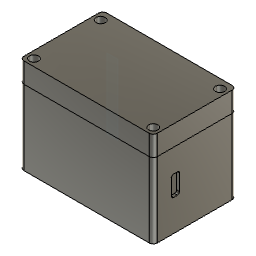
ESP32 Tally Case (Autodesk Fusion 360 design; units mm, degrees)
Autodesk Fusion 360 part; units mm, degrees
sketch "Sketch1" plane through (0, 0, 0) normal (0, 0, 1) x (1, 0, 0)
  line L0 (0, 0) -> (62, 0)
  line L1 (62, 0) -> (62, 39)
  line L2 (62, 39) -> (0, 39)
  line L3 (0, 39) -> (0, 0)
  line L4 (0, 0) -> (5, 0) construction
  line L5 (5, 0) -> (5, 5) construction
  line L6 (5, 5) -> (0, 5) construction
  line L7 (0, 5) -> (0, 0) construction
  line L8 (5, 5) -> (57, 5)
  line L9 (57, 5) -> (57, 34)
  line L10 (57, 34) -> (5, 34)
  line L11 (5, 34) -> (5, 5)
  dimension "d3" = 39
  dimension "d4" = 62
  dimension "d5" = 5
  dimension "d6" = 5
  dimension "d7" = 52
  dimension "d8" = 29
  constraint horizontal L0
  constraint vertical L1
  constraint horizontal L2
  constraint vertical L3
  constraint coincident L0.start L3.end
  constraint horizontal L4
  constraint vertical L5
  constraint horizontal L6
  constraint vertical L7
  constraint horizontal L8
  constraint vertical L9
  constraint horizontal L10
  constraint vertical L11
  measures "d3" distance of L0.start L2.end
  measures "d4" distance of L0.start L0.end
  measures "d5" distance of L0.start L4.end
  measures "d6" distance of L0.start L6.end
  measures "d7" distance of L5.end L8.end
  measures "d8" distance of L5.end L10.end
extrude "Extrude1" add sketch "Sketch1" along normal blind 8 contours L0 L1 L2 L3 | L8 L9 L10 L11 makes body 1
extrude "Extrude2" add sketch "Sketch1" along normal blind 23 bodies 1
sketch "Sketch2" plane through (0, 0, 23) normal (0, 0, 1) x (-1, 0, 0)
  line L0 (-5, -5) -> (-5, -34)
  line L1 (-5, -34) -> (-57, -34)
  line L2 (-57, -34) -> (-57, -5)
  line L3 (-57, -5) -> (-5, -5)
  line L4 (0, -39) -> (0, 0)
  line L5 (0, 0) -> (-62, 0)
  line L6 (-62, 0) -> (-62, -39)
  line L7 (-62, -39) -> (0, -39)
  line L8 (-31, -34) -> (-10.5, -34)
  line L9 (-31, -34) -> (-51.5, -34)
  line L10 (-62, -39) -> (-62, -37) construction
  line L11 (-62, -37) -> (0, -37) construction
  line L12 (-51.5, -34) -> (-10.5, -34)
  line L13 (-10.5, -34) -> (-10.5, -37)
  line L14 (-10.5, -37) -> (-51.5, -37)
  line L15 (-51.5, -37) -> (-51.5, -34)
  dimension "d13" = 20.5
  dimension "d14" = 20.5
  dimension "d15" = 2
  constraint midpoint L1 L8.start
  constraint parallel L1 L8
  constraint parallel L1 L9
  constraint coincident L6.end L7.start
  constraint perpendicular L7 L10
  constraint coincident L4 L11.end
  constraint perpendicular L4 L11
  constraint horizontal L12
  constraint vertical L13
  constraint horizontal L14
  constraint vertical L15
  constraint coincident L11 L13.end
  measures "d13" distance of L8.start L8.end
  measures "d14" distance of L8.start L9.end
  measures "d15" distance of L6.end L10.end
extrude "Extrude3" add sketch "Sketch2" along normal blind 6 bodies 1
sketch "Sketch3" plane through (0, 0, 29) normal (0, 0, 1) x (-1, 0, 0)
  line L0 (-10.5, -37) -> (-51.5, -37)
  line L1 (-51.5, -37) -> (-51.5, -34)
  line L2 (-51.5, -34) -> (-57, -34)
  line L3 (-57, -34) -> (-57, -5)
  line L4 (-57, -5) -> (-5, -5)
  line L5 (-5, -5) -> (-5, -34)
  line L6 (-5, -34) -> (-10.5, -34)
  line L7 (-10.5, -34) -> (-10.5, -37)
  line L8 (-62, -39) -> (0, -39)
  line L9 (0, -39) -> (0, 0)
  line L10 (0, 0) -> (-62, 0)
  line L11 (-62, 0) -> (-62, -39)
  line L12 (-51.5, -37) -> (-51.5, -39)
  line L13 (-10.5, -37) -> (-10.5, -39)
  constraint coincident L0.end L1.start
  constraint coincident L8 L12.end
  constraint perpendicular L8 L12
  constraint coincident L0.start L7.end
  constraint coincident L8 L13.end
  constraint perpendicular L8 L13
extrude "Extrude4" add sketch "Sketch3" along normal blind 29 contours L1 L2 L3 L4 L5 L6 L7 L8 L9 L10 L11 L12 L13 bodies 1
sketch "Sketch4" plane through (51.5, 0, 0) normal (-1, 0, 0) x (0, -1, 0)
  line L0 (-37, 23) -> (-34, 23)
  line L1 (-34, 23) -> (-34, 58)
  line L2 (-34, 58) -> (-39, 58)
  line L3 (-39, 58) -> (-39, 29)
  line L4 (-39, 29) -> (-37, 29)
  line L5 (-37, 29) -> (-37, 23)
  line L6 (-37, 29) -> (-37, 58)
  constraint coincident L4.end L5.start
  constraint coincident L2 L6.end
  constraint perpendicular L2 L6
sketch "Sketch5" plane through (10.5, 0, 0) normal (1, 0, 0) x (0, 1, 0)
  line L0 (34, 23) -> (37, 23)
  line L1 (37, 23) -> (37, 29)
  line L2 (37, 29) -> (39, 29)
  line L3 (39, 29) -> (39, 58)
  line L4 (39, 58) -> (34, 58)
  line L5 (34, 58) -> (34, 23)
  line L6 (37, 29) -> (37, 58)
  constraint coincident L1.end L2.start
  constraint coincident L4 L6.end
  constraint perpendicular L4 L6
extrude "Extrude5" add sketch "Sketch4" along normal blind 2.5 contours L2 L3 L4 L6 bodies 1
extrude "Extrude6" add sketch "Sketch5" along normal blind 2.5 contours L2 L3 L4 L6 bodies 1
extrude "Extrude7" add 1 faces at (20.6667, 0, 19.3333) along direction (0, -1, 0) blind 2 on bodies 1 bodies 1
extrude "Extrude8" add 1 faces at (62, 25.3333, 38.6667) along direction (1, 0, 0) blind 2 on bodies 1 bodies 1
extrude "Extrude9" add 1 faces at (0, 25.3333, 38.6667) along direction (-1, 0, 0) blind 2 on bodies 1 bodies 1
ref_plane "WorkPlane1" through (0, 0, 23) normal (0, 0, 1) x (1, 0, 0)
split "Split1" by plane through (0, 0, 23) normal (0, 0, 1) bodies 1 makes body 2 at (42, -2, 46.3333)
extrude "Extrude10" add 1 faces at (37, 38.3333, 29) along direction (0, 0, 1) blind 5 on bodies 2 bodies 2
sketch "Sketch6" plane through (13, 0, 0) normal (1, 0, 0) x (0, 1, 0)
  line L0 (37, 34) -> (39, 34)
  line L1 (39, 34) -> (39, 58)
  line L2 (39, 58) -> (37, 58)
  line L3 (37, 58) -> (37, 34)
  line L4 (37, 58) -> (39, 58)
  line L5 (39, 58) -> (39, 51)
  line L6 (39, 51) -> (37, 51)
  line L7 (37, 51) -> (37, 58)
  dimension "d33" = 7
  constraint horizontal L4
  constraint vertical L5
  constraint horizontal L6
  constraint vertical L7
  constraint coincident L2.end L3.start
  measures "d33" distance of L2.end L6.end
extrude "Extrude11" add sketch "Sketch6" along normal blind 40 contours L1 L2 L3 L4 L5 L6 L7 bodies 2
sketch "Sketch7" plane through (0, 34, 0) normal (0, -1, 0) x (1, 0, 0)
  line L0 (5, 23) -> (10.5, 23)
  line L1 (10.5, 23) -> (10.5, 58)
  line L2 (10.5, 58) -> (5, 58)
  line L3 (5, 58) -> (5, 23)
move_body "Move1" bodies 2 to x (1, 0, 0) y (0, 1, 0) z (0, 0, 1) at (0, 0, 2)
extrude "Extrude12" add 1 faces at (39.6667, 0.3333, 25) along direction (0, 0, -1) blind 2 on bodies 2 bodies 2
sketch "Sketch8" plane through (10.5, 0, 0) normal (1, 0, 0) x (0, 1, 0)
  line L0 (37, 23) -> (37, 60)
  line L1 (37, 60) -> (34, 60)
  line L2 (34, 60) -> (34, 23)
  line L3 (34, 23) -> (37, 23)
  line L4 (34, 23) -> (37, 23)
  line L5 (37, 23) -> (37, 25)
  line L6 (37, 25) -> (34, 25)
  line L7 (34, 25) -> (34, 23)
  dimension "d38" = 2
  constraint horizontal L4
  constraint vertical L5
  constraint horizontal L6
  constraint vertical L7
  measures "d38" distance of L2.end L6.end
extrude "Extrude13" add sketch "Sketch8" along normal blind 41 contours L0 L2 L3 L4 L5 L6 L7 bodies 2
sketch "Sketch9" plane through (0, 34, 0) normal (0, -1, 0) x (1, 0, 0)
  line L0 (10.5, 25) -> (10.5, 60)
  line L1 (10.5, 60) -> (5, 60)
  line L2 (5, 60) -> (5, 23)
  line L3 (5, 23) -> (57, 23)
  line L4 (57, 23) -> (57, 60)
  line L5 (57, 60) -> (51.5, 60)
  line L6 (51.5, 60) -> (51.5, 25)
  line L7 (51.5, 25) -> (10.5, 25)
extrude "Extrude14" add sketch "Sketch9" along normal blind 2 bodies 2
extrude "Extrude15" add 1 faces at (55.1667, 32, 36) along direction (0, -1, 0) blind 2 on bodies 2 bodies 2
sketch "Sketch10" plane through (0, 0, 25) normal (0, 0, 1) x (-1, 0, 0)
  line L0 (-10.5, -37) -> (-10.5, -30)
  line L1 (-10.5, -30) -> (-51.5, -30)
  line L2 (-51.5, -30) -> (-51.5, -37)
  line L3 (-51.5, -37) -> (-10.5, -37)
  line L4 (-51.5, -30) -> (-10.5, -30)
  line L5 (-10.5, -30) -> (-10.5, -32)
  line L6 (-10.5, -32) -> (-51.5, -32)
  line L7 (-51.5, -32) -> (-51.5, -30)
  dimension "d45" = 41
  dimension "d46" = 2
  constraint horizontal L4
  constraint vertical L5
  constraint horizontal L6
  constraint vertical L7
  constraint coincident L1.end L2.start
  measures "d45" distance of L1.end L0.end
  measures "d46" distance of L1.end L6.end
extrude "Extrude16" add sketch "Sketch10" along normal blind 25 contours L0 L1 L2 L4 L5 L6 L7 bodies 2
extrude "Extrude17" add 2 faces at (22.3333, 0.3333, 60) (37, 38.3333, 60) along direction (0, 0, 1) blind 2 separate body on bodies 2 makes body 3
extrude "Extrude18" cut 2 faces at (55.1667, 30, 61.3333) (8.6667, 30, 60.6667) along direction (0, 1, 0) blind 2 on bodies 3 bodies 3
extrude "Extrude19" add 1 faces at (51.5, 35.3333, 61.3333) along direction (-1, 0, 0) blind 41 on bodies 3 bodies 3
extrude "Extrude20" add 3 faces at (37, 33.6667, 62) (22.3333, 0.3333, 62) (37, 38.3333, 62) along direction (0, 0, 1) blind 6 on bodies 3 bodies 3
sketch "Sketch11" plane through (0, 0, 68) normal (0, 0, 1) x (-1, 0, 0)
  line L0 (-64, -39) -> (2, -39)
  line L1 (2, -39) -> (2, 2)
  line L2 (2, 2) -> (-64, 2)
  line L3 (-64, 2) -> (-64, -39)
  line L4 (-5, -32) -> (-57, -32)
  line L5 (-57, -32) -> (-57, -5)
  line L6 (-57, -5) -> (-5, -5)
  line L7 (-5, -5) -> (-5, -32)
  line L8 (-5, -32) -> (-5, -39) construction
  line L9 (-5, -5) -> (-5, 2) construction
  line L10 (-5, -5) -> (2, -5) construction
  line L11 (-57, -5) -> (-57, 2) construction
  line L12 (-57, -5) -> (-64, -5) construction
  line L13 (-57, -32) -> (-64, -32) construction
  line L14 (-57, -32) -> (-57, -39) construction
  line L15 (-5, -32) -> (2, -32) construction
  line L16 (-5, 2) -> (-7, 2) construction
  line L17 (-57, 2) -> (-55, 2) construction
  line L18 (-5, 2) -> (-5, 0) construction
  line L19 (-5, -39) -> (-5, -37) construction
  line L20 (-55, 2) -> (-55, 0) construction
  line L21 (-5, -37) -> (-7, -37)
  line L22 (-7, -37) -> (-55, -37)
  line L23 (-55, -37) -> (-55, 0)
  line L24 (-55, 0) -> (-7, 0)
  line L25 (-7, 0) -> (-7, -37)
  line L26 (-64, -5) -> (-62, -5) construction
  line L27 (-62, -5) -> (-62, -7) construction
  line L28 (-62, -7) -> (-64, -7) construction
  line L29 (-64, -7) -> (-64, -5) construction
  line L30 (2, -32) -> (0, -32)
  line L31 (0, -32) -> (0, -30)
  line L32 (0, -30) -> (2, -30)
  line L33 (2, -30) -> (2, -32)
  line L34 (0, -30) -> (-62, -30)
  line L35 (-62, -30) -> (-62, -7)
  line L36 (-62, -7) -> (0, -7)
  line L37 (0, -7) -> (0, -30)
  dimension "d57" = 2
  dimension "d58" = 2
  dimension "d59" = 2
  dimension "d60" = 2
  dimension "d61" = 2
  dimension "d62" = 2
  dimension "d63" = 2
  dimension "d64" = 2
  dimension "d65" = 2
  dimension "d66" = 2
  constraint coincident L4.start L7.end
  constraint coincident L0 L8.end
  constraint perpendicular L0 L8
  constraint coincident L6.end L7.start
  constraint coincident L2 L9.end
  constraint perpendicular L2 L9
  constraint coincident L1 L10.end
  constraint perpendicular L1 L10
  constraint coincident L5.end L6.start
  constraint coincident L2 L11.end
  constraint perpendicular L2 L11
  constraint coincident L3 L12.end
  constraint perpendicular L3 L12
  constraint coincident L4.end L5.start
  constraint coincident L3 L13.end
  constraint perpendicular L3 L13
  constraint coincident L0 L14.end
  constraint perpendicular L0 L14
  constraint coincident L1 L15.end
  constraint perpendicular L1 L15
  constraint perpendicular L9 L16
  constraint perpendicular L11 L17
  constraint perpendicular L16 L18
  constraint perpendicular L0 L19
  constraint perpendicular L17 L20
  constraint perpendicular L19 L21
  constraint horizontal L22
  constraint vertical L23
  constraint horizontal L24
  constraint vertical L25
  constraint horizontal L26
  constraint vertical L27
  constraint horizontal L28
  constraint vertical L29
  constraint horizontal L30
  constraint vertical L31
  constraint horizontal L32
  constraint vertical L33
  constraint horizontal L34
  constraint vertical L35
  constraint horizontal L36
  constraint vertical L37
  measures "d57" distance of L9.end L16.end
  measures "d58" distance of L11.end L17.end
  measures "d59" distance of L9.end L18.end
  measures "d60" distance of L8.end L19.end
  measures "d61" distance of L17.end L20.end
  measures "d62" distance of L19.end L21.end
  measures "d63" distance of L12.end L26.end
  measures "d64" distance of L12.end L28.end
  measures "d65" distance of L15.end L30.end
  measures "d66" distance of L15.end L32.end
extrude "Extrude21" cut sketch "Sketch11" against normal blind 22 contours L7 L34 L36 L37 | L4 L22 L23 L25 | L6 L23 L24 L25 | L5 L34 L35 L36 bodies 3
sketch "Sketch12" plane through (0, 37, 0) normal (0, -1, 0) x (1, 0, 0)
  line L0 (7, 60) -> (55, 60)
  line L1 (55, 60) -> (55, 68)
  line L2 (55, 68) -> (7, 68)
  line L3 (7, 68) -> (7, 60)
  line L4 (31, 60) -> (27, 60)
  line L5 (31, 60) -> (35, 60)
  line L6 (35, 60) -> (27, 60)
  line L7 (27, 60) -> (27, 61)
  line L8 (27, 61) -> (35, 61)
  line L9 (35, 61) -> (35, 60)
  dimension "d69" = 4
  dimension "d70" = 4
  dimension "d71" = 8
  dimension "d72" = 1
  constraint midpoint L0 L4.start
  constraint parallel L0 L4
  constraint parallel L0 L5
  constraint horizontal L6
  constraint vertical L7
  constraint horizontal L8
  constraint vertical L9
  measures "d69" distance of L4.start L4.end
  measures "d70" distance of L4.start L5.end
  measures "d71" distance of L5.end L4.end
  measures "d72" distance of L5.end L8.end
extrude "Extrude22" add sketch "Sketch12" along normal blind 37 contours L0 L4 L5 L6 L7 L8 L9 bodies 3
sketch "Sketch13" plane through (0, 0, 68) normal (0, 0, 1) x (-1, 0, 0)
  line L0 (-57, -30) -> (-62, -30)
  line L1 (-62, -30) -> (-62, -7)
  line L2 (-62, -7) -> (-57, -7)
  line L3 (-57, -7) -> (-57, -5)
  line L4 (-57, -5) -> (-55, -5)
  line L5 (-55, -5) -> (-55, 0)
  line L6 (-55, 0) -> (-7, 0)
  line L7 (-7, 0) -> (-7, -5)
  line L8 (-7, -5) -> (-5, -5)
  line L9 (-5, -5) -> (-5, -7)
  line L10 (-5, -7) -> (0, -7)
  line L11 (0, -7) -> (0, -30)
  line L12 (0, -30) -> (-5, -30)
  line L13 (-5, -30) -> (-5, -32)
  line L14 (-5, -32) -> (-7, -32)
  line L15 (-7, -32) -> (-7, -37)
  line L16 (-7, -37) -> (-55, -37)
  line L17 (-55, -37) -> (-55, -32)
  line L18 (-55, -32) -> (-57, -32)
  line L19 (-57, -32) -> (-57, -30)
  line L20 (-64, -39) -> (2, -39)
  line L21 (2, -39) -> (2, 2)
  line L22 (2, 2) -> (-64, 2)
  line L23 (-64, 2) -> (-64, -39)
extrude "Extrude23" add sketch "Sketch13" along normal blind 2 contours L0 L1 L2 L3 L4 L5 L6 L7 L8 L9 L10 L11 L12 L13 L14 L15 L16 L17 L18 L19 | L20 L21 L22 L23 bodies 3
sketch "Sketch14" plane through (0, 0, 23) normal (0, 0, -1) x (1, 0, 0)
  line L0 (57, -5) -> (57, -30)
  line L1 (57, -30) -> (5, -30)
  line L2 (5, -30) -> (5, -5)
  line L3 (5, -5) -> (57, -5)
  line L4 (64, -39) -> (64, 2)
  line L5 (64, 2) -> (-2, 2)
  line L6 (-2, 2) -> (-2, -39)
  line L7 (-2, -39) -> (64, -39)
  line L8 (64, -39) -> (57, -30) construction
  line L9 (64, 2) -> (57, -5) construction
  line L10 (5, -30) -> (-2, -39) construction
  line L11 (-2, 2) -> (5, -5) construction
  circle A0 centre (1.5, -34.5) radius 2.25
  circle A1 centre (1.5, -1.5) radius 2.25
  circle A2 centre (60.5, -1.5) radius 2.25
  circle A3 centre (60.5, -34.5) radius 2.25
  dimension "d77" = 4.5
  dimension "d78" = 4.5
  dimension "d79" = 4.5
  dimension "d80" = 4.5
  constraint coincident L4.start L7.end
  constraint coincident L0.end L1.start
  constraint coincident L4.end L5.start
  constraint coincident L0.start L3.end
  constraint coincident L1.end L2.start
  constraint coincident L6.end L7.start
  constraint coincident L5.end L6.start
  constraint coincident L2.end L3.start
  constraint midpoint L10 A0.centre
  constraint midpoint L11 A1.centre
  constraint midpoint L9 A2.centre
  constraint midpoint L8 A3.centre
  measures "d77" diameter of A0
  measures "d78" diameter of A1
  measures "d79" diameter of A2
  measures "d80" diameter of A3
extrude "Extrude24" cut sketch "Sketch14" along normal blind 25 and the other way blind 50 contours A0 | A1 | A2 | A3 bodies 1 2 3
fillet "Fillet1" radius 2 12 edges at (64, 39, 11.5) (64, -2, 11.5) (-2, 39, 11.5) (-2, -2, 11.5) (64, 39, 41.5) (64, -2, 41.5) (-2, 39, 41.5) (-2, -2, 41.5) (64, 39, 65) (64, -2, 65) (-2, 39, 65) (-2, -2, 65) on bodies 1 2 3
sketch "Sketch15" plane through (0, 0, 0) normal (0, 0, -1) x (1, 0, 0)
  arc A0 (0, 2) -> (-2, 0) centre (0, 0) ccw
  line L0 (-2, 0) -> (-2, -37)
  arc A1 (-2, -37) -> (0, -39) centre (0, -37) ccw
  line L1 (0, -39) -> (62, -39)
  arc A2 (62, -39) -> (64, -37) centre (62, -37) ccw
  line L2 (64, -37) -> (64, 0)
  arc A3 (64, 0) -> (62, 2) centre (62, 0) ccw
  line L3 (62, 2) -> (0, 2)
  circle A4 centre (60.5, -1.5) radius 2.25
  circle A5 centre (1.5, -34.5) radius 2.25
  circle A6 centre (60.5, -34.5) radius 2.25
  circle A7 centre (1.5, -1.5) radius 2.25
  line L4 (31, -39) -> (31, 2)
  line L5 (38.5, -11) -> (23.5, -11) construction
  line L6 (23.5, -11) -> (23.5, -26) construction
  line L7 (23.5, -26) -> (38.5, -26) construction
  line L8 (38.5, -26) -> (38.5, -11) construction
  line L9 (38.5, -11) -> (23.5, -26) construction
  line L10 (23.5, -11) -> (38.5, -26) construction
  line L11 (31, -18.5) -> (38.5, -26) construction
  line L12 (23.5, -11) -> (31, -18.5) construction
  circle A8 centre (27.25, -14.75) radius 2.25
  circle A9 centre (34.75, -22.25) radius 2.25
  point P0 (31, -18.5)
  dimension "d87" = 15
  dimension "d88" = 15
  dimension "d90" = 4.5
  dimension "d91" = 4.5
  constraint midpoint L1 L4.start
  constraint midpoint L3 L4.end
  constraint horizontal L5
  constraint perpendicular L5 L6
  constraint parallel L5 L7
  constraint parallel L6 L8
  constraint coincident L9 P0
  constraint coincident L10 P0
  constraint midpoint L4 P0
  constraint coincident P0 L11.start
  constraint midpoint L12 A8.centre
  constraint midpoint L11 A9.centre
  measures "d87" distance of L6.end L7.end
  measures "d88" distance of L5.end L6.end
  measures "d90" diameter of A8
  measures "d91" diameter of A9
extrude "Extrude25" cut sketch "Sketch15" against normal blind 4 contours A8 | A9 bodies 1
sketch "Sketch16" plane through (5, 0, 0) normal (1, 0, 0) x (0, 1, 0)
  line L0 (34, 23) -> (5, 23)
  line L1 (5, 23) -> (5, 8)
  line L2 (5, 8) -> (34, 8)
  line L3 (34, 8) -> (34, 23)
  line L4 (19.5, 8) -> (12, 8)
  line L5 (19.5, 8) -> (27, 8)
  line L6 (12, 8) -> (27, 8)
  line L7 (27, 8) -> (27, 16)
  line L8 (27, 16) -> (12, 16)
  line L9 (12, 16) -> (12, 8)
  dimension "d94" = 7.5
  dimension "d95" = 7.5
  dimension "d96" = 8
  constraint midpoint L2 L4.start
  constraint parallel L2 L4
  constraint parallel L2 L5
  constraint horizontal L6
  constraint vertical L7
  constraint horizontal L8
  constraint vertical L9
  measures "d94" distance of L4.start L4.end
  measures "d95" distance of L4.start L5.end
  measures "d96" distance of L4.end L8.end
extrude "Extrude26" cut sketch "Sketch16" against normal blind 36 contours L2 L4 L5 L6 L7 L8 L9 bodies 1
fillet "Fillet2" radius 2.5 4 edges at (1.5, 27, 8) (1.5, 12, 8) (1.5, 12, 16) (1.5, 27, 16) on bodies 1
fillet "Fillet3" radius 1.5 8 edges at (-2, 12.7322, 15.2678) (-2, 12, 12) (-2, 12.7322, 8.7322) (-2, 19.5, 8) (-2, 26.2678, 8.7322) (-2, 27, 12) (-2, 26.2678, 15.2678) (-2, 19.5, 16) on bodies 1
extrude "Extrude27" cut 1 faces at (57, 24.3333, 13) along direction (1, 0, 0) blind 0.5 on bodies 1 bodies 1
extrude "Extrude28" cut 1 faces at (5, 17.8333, 20.6667) along direction (-1, 0, 0) blind 0.5 on bodies 1 bodies 1
extrude "Extrude29" cut 1 faces at (39.8333, 34, 13) along direction (0, 1, 0) blind 0.5 on bodies 1 bodies 1
extrude "Extrude30" cut 1 faces at (39.8333, 5, 18) along direction (0, -1, 0) blind 0.5 on bodies 1 bodies 1
extrude "Extrude31" cut 1 faces at (10.5, 35.3333, 45) along direction (-1, 0, 0) blind 0.5 on bodies 2 bodies 2
extrude "Extrude32" cut 1 faces at (51.5, 35.3333, 45) along direction (1, 0, 0) blind 0.5 on bodies 2 bodies 2
extrude "Extrude33" cut 1 faces at (38, 32, 33.3333) along direction (0, -1, 0) blind 0.5 on bodies 2 bodies 2
copy_body "Body->Comp1" bodies 3 removing the originals makes body 4 in component "Component"
copy_body "Body->Comp2" bodies 2 removing the originals makes body 5 in component "Component'"
extrude "Extrude1'" add 1 faces at (38, 31.5, 33.3333) along direction (0, 1, 0) blind 0.5 on bodies 5 bodies 5 in component "Component'"
sketch "Sketch17" plane through (0, 0, 36) normal (0, 0, 1) x (-1, 0, 0)
  line L0 (-13, -39) -> (-13, -37)
  line L1 (-13, -37) -> (-49, -37)
  line L2 (-49, -37) -> (-49, -39)
  line L3 (-49, -39) -> (-13, -39)
  line L4 (-31, -39) -> (-46, -39)
  line L5 (-31, -39) -> (-16, -39)
  line L6 (-16, -39) -> (-13, -39)
  line L7 (-13, -39) -> (-13, -37)
  line L8 (-13, -37) -> (-16, -37)
  line L9 (-16, -37) -> (-16, -39)
  line L10 (-46, -39) -> (-49, -39)
  line L11 (-49, -39) -> (-49, -37)
  line L12 (-49, -37) -> (-46, -37)
  line L13 (-46, -37) -> (-46, -39)
  dimension "d119" = 15
  dimension "d120" = 15
  constraint midpoint L3 L4.start
  constraint parallel L3 L4
  constraint parallel L3 L5
  constraint horizontal L6
  constraint vertical L7
  constraint horizontal L8
  constraint vertical L9
  constraint coincident L0.end L1.start
  constraint horizontal L10
  constraint vertical L11
  constraint horizontal L12
  constraint vertical L13
  constraint coincident L1.end L2.start
  measures "d119" distance of L4.start L4.end
  measures "d120" distance of L4.start L5.end
extrude "Extrude2'" add sketch "Sketch17" along normal blind 17 contours L0 L1 L3 L6 L7 L8 L9 | L1 L2 L3 L10 L11 L12 L13 bodies 5 in component "Component'"
sketch "Sketch18" plane through (0, 5, 0) normal (0, 1, 0) x (-1, 0, 0)
  line L0 (-5, 23) -> (-5, 60)
  line L1 (-5, 60) -> (-57, 60)
  line L2 (-57, 60) -> (-57, 23)
  line L3 (-57, 23) -> (-5, 23)
  line L4 (-57, 23) -> (-5, 23)
  line L5 (-5, 23) -> (-5, 29)
  line L6 (-5, 29) -> (-57, 29)
  line L7 (-57, 29) -> (-57, 23)
  dimension "d123" = 6
  constraint horizontal L4
  constraint vertical L5
  constraint horizontal L6
  constraint vertical L7
  constraint coincident L2.end L3.start
  measures "d123" distance of L2.end L6.end
extrude "Extrude3'" add sketch "Sketch18" along normal blind 25 contours L0 L2 L3 L4 L5 L6 L7 bodies 5 in component "Component'"
extrude "Extrude4'" add 1 faces at (39.6667, 5, 49.6667) along direction (0, 1, 0) blind 2 on bodies 5 bodies 5 in component "Component'"
extrude "Extrude5'" cut 1 faces at (57, 22.3333, 49.6667) along direction (1, 0, 0) blind 5.5 on bodies 5 bodies 5 in component "Component'"
extrude "Extrude6'" add 1 faces at (5, 22.3333, 49.6667) along direction (1, 0, 0) blind 5.5 on bodies 5 bodies 5 in component "Component'"
sketch "Sketch19" plane through (62.5, 0, 0) normal (-1, 0, 0) x (0, -1, 0)
  line L0 (-7, 29) -> (-7, 60)
  line L1 (-7, 60) -> (-30, 60)
  line L2 (-30, 60) -> (-30, 29)
  line L3 (-30, 29) -> (-7, 29)
  line L4 (-7, 29) -> (-7, 58)
  line L5 (-7, 43.5) -> (-14, 43.5) construction
  line L6 (-7, 43.5) -> (-7, 48.5)
  line L7 (-7, 43.5) -> (-7, 38.5)
  line L8 (-7, 38.5) -> (-11, 38.5)
  line L9 (-11, 38.5) -> (-11, 48.5)
  line L10 (-11, 48.5) -> (-7, 48.5)
  line L11 (-7, 48.5) -> (-7, 38.5)
  dimension "d132" = 29
  dimension "d133" = 5
  dimension "d134" = 5
  dimension "d135" = 4
  constraint coincident L0.start L3.end
  constraint perpendicular L3 L4
  constraint midpoint L4 L5.start
  constraint perpendicular L0 L5
  constraint perpendicular L5 L6
  constraint coincident L0 L7.end
  constraint perpendicular L5 L7
  constraint horizontal L8
  constraint vertical L9
  constraint horizontal L10
  constraint vertical L11
  measures "d132" distance of L0.start L4.end
  measures "d133" distance of L5.start L6.end
  measures "d134" distance of L5.start L7.end
  measures "d135" distance of L7.end L8.end
extrude "Extrude7'" cut sketch "Sketch19" against normal blind 10 contours L0 L4 L6 L7 L8 L9 L10 L11 bodies 5 in component "Component'"
fillet "Fillet1'" radius 1 4 edges at (63.25, 7, 38.5) (63.25, 11, 38.5) (63.25, 7, 48.5) (63.25, 11, 48.5) on bodies 5 in component "Component'"
sketch "Sketch20" plane through (0, 0, 23) normal (0, 0, -1) x (1, 0, 0)
  arc A0 (0, 2) -> (-2, 0) centre (0, 0) ccw
  line L0 (-2, 0) -> (-2, -37)
  arc A1 (-2, -37) -> (0, -39) centre (0, -37) ccw
  line L1 (0, -39) -> (62, -39)
  arc A2 (62, -39) -> (64, -37) centre (62, -37) ccw
  line L2 (64, -37) -> (64, 0)
  arc A3 (64, 0) -> (62, 2) centre (62, 0) ccw
  line L3 (62, 2) -> (0, 2)
  circle A4 centre (60.5, -1.5) radius 2.25
  circle A5 centre (1.5, -34.5) radius 2.25
  circle A6 centre (60.5, -34.5) radius 2.25
  circle A7 centre (1.5, -1.5) radius 2.25
  line L4 (31, 2) -> (31, -39) construction
  line L5 (26, -23.5) -> (36, -23.5) construction
  line L6 (36, -23.5) -> (36, -13.5) construction
  line L7 (36, -13.5) -> (26, -13.5) construction
  line L8 (26, -13.5) -> (26, -23.5) construction
  line L9 (26, -23.5) -> (36, -13.5) construction
  line L10 (36, -23.5) -> (26, -13.5) construction
  line L11 (31, -18.5) -> (36, -23.5) construction
  line L12 (26.3241, -13.8241) -> (31, -18.5) construction
  circle A8 centre (33.5, -21) radius 2.25
  circle A9 centre (28.6621, -16.1621) radius 2.25
  point P0 (31, -18.5)
  dimension "d140" = 10
  dimension "d141" = 10
  dimension "d142" = 4.5
  dimension "d143" = 4.5
  constraint midpoint L3 L4.start
  constraint midpoint L1 L4.end
  constraint horizontal L5
  constraint perpendicular L5 L6
  constraint parallel L5 L7
  constraint parallel L6 L8
  constraint coincident L9 P0
  constraint coincident L10 P0
  constraint midpoint L4 P0
  constraint coincident P0 L11.start
  constraint coincident L10 L12.start
  constraint perpendicular L9 L12
  constraint midpoint L11 A8.centre
  constraint midpoint L12 A9.centre
  measures "d140" distance of L6.end L7.end
  measures "d141" distance of L5.end L6.end
  measures "d142" diameter of A8
  measures "d143" diameter of A9
extrude "Extrude8'" cut sketch "Sketch20" against normal blind 4 contours A8 | A9 bodies 5 in component "Component'"
delete_body "RemoveBody4" bodies 1
sketch "Sketch21" plane through (-2, 0, 0) normal (-1, 0, 0) x (0, -1, 0)
  line L0 (0, 23) -> (0, 60)
  line L1 (0, 60) -> (-37, 60)
  line L2 (-37, 60) -> (-37, 23)
  line L3 (-37, 23) -> (0, 23)
  line L4 (-18.5, 23) -> (-18.5, 60) construction
  line L5 (-13.5, 46.5) -> (-23.5, 46.5)
  line L6 (-23.5, 46.5) -> (-23.5, 36.5)
  line L7 (-23.5, 36.5) -> (-13.5, 36.5)
  line L8 (-13.5, 36.5) -> (-13.5, 46.5)
  line L9 (-13.5, 46.5) -> (-23.5, 36.5) construction
  line L10 (-23.5, 46.5) -> (-13.5, 36.5) construction
  line L11 (-18.5, 41.5) -> (-23.5, 46.5) construction
  line L12 (-18.5, 41.5) -> (-13.5, 36.5) construction
  circle A0 centre (-16, 39) radius 2.25
  circle A1 centre (-21, 44) radius 2.25
  point P0 (-18.5, 41.5)
  dimension "d146" = 10
  dimension "d147" = 10
  dimension "d148" = 4.5
  dimension "d149" = 4.5
  constraint midpoint L3 L4.start
  constraint midpoint L1 L4.end
  constraint horizontal L5
  constraint perpendicular L5 L6
  constraint parallel L5 L7
  constraint parallel L6 L8
  constraint coincident L9 P0
  constraint coincident L10 P0
  constraint midpoint L4 P0
  constraint coincident P0 L11.start
  constraint midpoint L12 A0.centre
  constraint midpoint L11 A1.centre
  measures "d146" distance of L6.end L7.end
  measures "d147" distance of L5.end L6.end
  measures "d148" diameter of A0
  measures "d149" diameter of A1
extrude "Extrude9'" cut sketch "Sketch21" against normal blind 11 contours A0 | A1 bodies 5 in component "Component'"
component "Component" placed x (1, 0, 0) y (0, 1, 0) z (0, 0, 1) at (0, 0, 0)
component "Component'" placed x (1, 0, 0) y (0, 1, 0) z (0, 0, 1) at (0, 0, 0)
equation "d3 = 29 mm + 5 mm + 5 mm"
equation "d4 = 52 mm + 5 mm + 5 mm"
equation "d11 = 15 mm + 8.00 mm"
equation "d13 = ( 41 / 2 ) * 1 mm"
equation "d14 = ( 41 / 2 ) * 1 mm"
equation "d18 = 34 mm - 5 mm"
equation "d30 = 8 mm + 15 mm"
